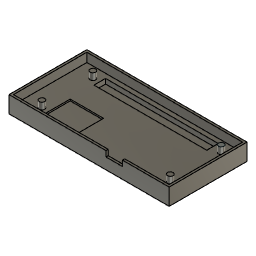
baseplate v7 (Autodesk Fusion 360 design; units mm, degrees)
Autodesk Fusion 360 part; units mm, degrees
sketch "Sketch1" plane through (0, 0, 0) normal (0, 0, 1) x (1, 0, 0)
  line L0 (0, 0) -> (70.5, 0)
  line L1 (70.5, 0) -> (70.5, 32)
  line L2 (70.5, 32) -> (0, 32)
  line L3 (0, 32) -> (0, 0)
  dimension "d1" = 70.5
  dimension "d2" = 32
  constraint horizontal L0
  constraint vertical L1
  constraint horizontal L2
  constraint vertical L3
  constraint coincident L0.start L3.end
  measures "d1" distance of L0.start L0.end
  measures "d2" distance of L0.start L2.end
extrude "Extrude1" add sketch "Sketch1" along normal blind 1.5
extrude "Extrude2" add 1 faces at (47, 32, 0.5) along direction (0, 1, 0) blind 1
extrude "Extrude3" add 1 faces at (23.5, 22, 1.5) along direction (0, 0, 1) blind 2
sketch "Sketch2" plane through (0, 0, 3.5) normal (0, 0, 1) x (-1, 0, 0)
  line L0 (0, -33) -> (0, 0)
  line L1 (0, 0) -> (-70.5, 0)
  line L2 (-70.5, 0) -> (-70.5, -33)
  line L3 (-70.5, -33) -> (0, -33)
  line L4 (-35.25, -33) -> (-35.25, -31)
  line L5 (-35.25, -31) -> (-35.25, -28.75)
  line L6 (-60.25, -26.5) -> (-10.25, -26.5)
  line L7 (-10.25, -26.5) -> (-10.25, -31)
  line L8 (-10.25, -31) -> (-60.25, -31)
  line L9 (-60.25, -31) -> (-60.25, -26.5)
  line L10 (-60.25, -26.5) -> (-10.25, -31) construction
  line L11 (-10.25, -26.5) -> (-60.25, -31) construction
  point P0 (-35.25, -28.75)
  dimension "d9" = 2
  dimension "d10" = 2.25
  dimension "d11" = 50
  dimension "d12" = 4.5
  constraint midpoint L3 L4.start
  constraint perpendicular L3 L4
  constraint perpendicular L3 L5
  constraint horizontal L6
  constraint perpendicular L6 L7
  constraint parallel L6 L8
  constraint parallel L7 L9
  constraint coincident L10 P0
  constraint coincident L11 P0
  constraint coincident P0 L5.end
  measures "d9" distance of L4.start L4.end
  measures "d10" distance of L4.end P0
  measures "d11" distance of L7.end L8.end
  measures "d12" distance of L6.end L7.end
extrude "Extrude4" cut sketch "Sketch2" against normal blind 2.2 contours L6 L7 L8 L9
extrude "Extrude5" cut 1 faces at (43.5833, 26.5, 2.7667) along direction (0, -1, 0) blind 0.7
extrude "Extrude6" cut 1 faces at (10.25, 27.5333, 2.7667) along direction (-1, 0, 0) blind 0.35
extrude "Extrude7" cut 1 faces at (60.25, 27.5333, 2.0333) along direction (1, 0, 0) blind 0.35
extrude "Extrude8" add 1 faces at (0, 22, 2.3333) along direction (-1, 0, 0) blind 1.5
extrude "Extrude9" add 1 faces at (22.5, 33, 1.1667) along direction (0, 1, 0) blind 1
extrude "Extrude10" add 1 faces at (46.5, 0, 1.1667) along direction (0, -1, 0) blind 1
sketch "Sketch3" plane through (0, 0, 3.5) normal (0, 0, 1) x (-1, 0, 0)
  line L0 (-60.6, -25.8) -> (-9.9, -25.8)
  line L1 (-9.9, -25.8) -> (-9.9, -31)
  line L2 (-9.9, -31) -> (-60.6, -31)
  line L3 (-60.6, -31) -> (-60.6, -25.8)
  line L4 (-70.5, 1) -> (-70.5, -34)
  line L5 (-70.5, -34) -> (1.5, -34)
  line L6 (1.5, -34) -> (1.5, 1)
  line L7 (1.5, 1) -> (-70.5, 1)
  line L8 (-10, -15) -> (-25, -15)
  line L9 (-25, -15) -> (-25, -3)
  line L10 (-25, -3) -> (-10, -3)
  line L11 (-10, -3) -> (-10, -15)
  constraint horizontal L8
  constraint vertical L9
  constraint horizontal L10
  constraint vertical L11
extrude "Extrude11" cut sketch "Sketch3" against normal blind 0.7 contours L8 L9 L10 L11
sketch "Sketch4" plane through (0, 0, 3.5) normal (0, 0, 1) x (-1, 0, 0)
  line L0 (-25, -15) -> (-25, -3)
  line L1 (-25, -3) -> (-10, -3)
  line L2 (-10, -3) -> (-10, -15)
  line L3 (-10, -15) -> (-25, -15)
  line L4 (-60.6, -25.8) -> (-9.9, -25.8)
  line L5 (-9.9, -25.8) -> (-9.9, -31)
  line L6 (-9.9, -31) -> (-60.6, -31)
  line L7 (-60.6, -31) -> (-60.6, -25.8)
  line L8 (-70.5, 1) -> (-70.5, -34)
  line L9 (-70.5, -34) -> (1.5, -34)
  line L10 (1.5, -34) -> (1.5, 1)
  line L11 (1.5, 1) -> (-70.5, 1)
  line L12 (1.5, -34) -> (-70.5, -34)
  line L13 (-70.5, -34) -> (-70.5, -33)
  line L14 (-70.5, -33) -> (1.5, -33)
  line L15 (1.5, -33) -> (1.5, -34)
  line L16 (1.5, 1) -> (0.5, 1)
  line L17 (0.5, 1) -> (0.5, -34)
  line L18 (0.5, -34) -> (1.5, -34)
  line L19 (1.5, -34) -> (1.5, 1)
  line L20 (1.5, 1) -> (-70.5, 1)
  line L21 (-70.5, 1) -> (-70.5, 0)
  line L22 (-70.5, 0) -> (1.5, 0)
  line L23 (1.5, 0) -> (1.5, 1)
  line L24 (-70.5, -34) -> (-69.5, -34)
  line L25 (-69.5, -34) -> (-69.5, 1)
  line L26 (-69.5, 1) -> (-70.5, 1)
  line L27 (-70.5, 1) -> (-70.5, -34)
  dimension "d29" = 1
  dimension "d30" = 1
  dimension "d31" = 1
  dimension "d32" = 1
  constraint horizontal L12
  constraint vertical L13
  constraint horizontal L14
  constraint vertical L15
  constraint coincident L9.end L10.start
  constraint horizontal L16
  constraint vertical L17
  constraint horizontal L18
  constraint vertical L19
  constraint coincident L10.end L11.start
  constraint horizontal L20
  constraint vertical L21
  constraint horizontal L22
  constraint vertical L23
  constraint horizontal L24
  constraint vertical L25
  constraint horizontal L26
  constraint vertical L27
  constraint coincident L8.end L9.start
  measures "d29" distance of L9.end L14.end
  measures "d30" distance of L10.end L16.end
  measures "d31" distance of L10.end L22.end
  measures "d32" distance of L8.end L24.end
extrude "Extrude12" add sketch "Sketch4" along normal blind 4 contours L8 L11 L20 L21 L22 L25 L26 L27 | L8 L14 L22 L25 L27 | L11 L17 L20 L22 L25 | L8 L9 L12 L13 L14 L24 L25 L27 | L10 L11 L16 L17 L19 L20 L22 L23 | L9 L12 L14 L17 L25 | L10 L14 L17 L19 L22 | L9 L10 L12 L14 L15 L17 L18 L19
sketch "Sketch5" plane through (0, 0, 3.5) normal (0, 0, 1) x (-1, 0, 0)
  line L0 (-69.5, -33) -> (0.5, -33)
  line L1 (0.5, -33) -> (0.5, 0)
  line L2 (0.5, 0) -> (-69.5, 0)
  line L3 (-69.5, 0) -> (-69.5, -33)
  line L4 (-25, -15) -> (-25, -3)
  line L5 (-25, -3) -> (-10, -3)
  line L6 (-10, -3) -> (-10, -15)
  line L7 (-10, -15) -> (-25, -15)
  line L8 (-60.6, -25.8) -> (-9.9, -25.8)
  line L9 (-9.9, -25.8) -> (-9.9, -31)
  line L10 (-9.9, -31) -> (-60.6, -31)
  line L11 (-60.6, -31) -> (-60.6, -25.8)
  line L12 (-70.5579, -29.7) -> (-66.2579, -29.7)
  circle A0 centre (-66.2579, -29.7) radius 1.375
  line L13 (-2, -34) -> (-2, -29.7)
  line L14 (1.461, -29.9433) -> (-5.539, -29.9433)
  circle A1 centre (-5.539, -29.9433) radius 1.375
  dimension "d36" = 4.3
  dimension "d37" = 2.75
  dimension "d38" = 4.3
  dimension "d39" = 7
  dimension "d40" = 2.75
  constraint perpendicular L3 L12
  constraint coincident L12.end A0.centre
  constraint perpendicular L0 L13
  constraint perpendicular L13 L14
  constraint coincident L14.end A1.centre
  measures "d36" distance of L12.start L12.end
  measures "d37" diameter of A0
  measures "d38" distance of L13.start L13.end
  measures "d39" distance of L14.start L14.end
  measures "d40" diameter of A1
extrude "Extrude13" add sketch "Sketch5" along normal blind 5 contours A0 | A1
sketch "Sketch6" plane through (0, -1, 0) normal (0, -1, 0) x (1, 0, 0)
  line L0 (-1.5, 0) -> (70.5, 0)
  line L1 (70.5, 0) -> (70.5, 7.5)
  line L2 (70.5, 7.5) -> (-1.5, 7.5)
  line L3 (-1.5, 7.5) -> (-1.5, 0)
  line L4 (70.5, 6.1254) -> (49.5, 6.1254)
  line L5 (49.5, 6.1254) -> (42.1, 6.1254)
  line L6 (42.1, 6.1254) -> (42.1, 7.5)
  line L7 (42.1, 7.5) -> (42.1, 8)
  line L8 (42.1, 8) -> (49.5, 8)
  line L9 (42.1, 8) -> (49.5, 8)
  line L10 (49.5, 8) -> (49.5, 5)
  line L11 (49.5, 5) -> (42.1, 5)
  line L12 (42.1, 5) -> (42.1, 8)
  dimension "d43" = 21
  dimension "d44" = 7.4
  dimension "d45" = 0.5
  dimension "d46" = 3
  constraint coincident L1 L4.start
  constraint perpendicular L1 L4
  constraint parallel L4 L5
  constraint coincident L2 L6.end
  constraint perpendicular L2 L6
  constraint vertical L7
  constraint perpendicular L7 L8
  constraint horizontal L9
  constraint vertical L10
  constraint horizontal L11
  constraint vertical L12
  measures "d43" distance of L4.start L4.end
  measures "d44" distance of L4.end L5.end
  measures "d45" distance of L6.end L7.end
  measures "d46" distance of L7.end L11.end
extrude "Extrude14" cut sketch "Sketch6" against normal blind 1 contours L2 L7 L8 L9 L10 L12 | L2 L5 L6 L10 L12 | L5 L10 L11 L12
sketch "Sketch7" plane through (0, 0, 3.5) normal (0, 0, 1) x (-1, 0, 0)
  circle A0 centre (-66.2579, -29.7) radius 1.375
  circle A1 centre (-5.539, -29.9433) radius 1.375
  line L0 (-69.5, -33) -> (0.5, -33)
  line L1 (0.5, -33) -> (0.5, 0)
  line L2 (0.5, 0) -> (-69.5, 0)
  line L3 (-69.5, 0) -> (-69.5, -33)
  line L4 (-25, -15) -> (-25, -3)
  line L5 (-25, -3) -> (-10, -3)
  line L6 (-10, -3) -> (-10, -15)
  line L7 (-10, -15) -> (-25, -15)
  line L8 (-60.6, -25.8) -> (-9.9, -25.8)
  line L9 (-9.9, -25.8) -> (-9.9, -31)
  line L10 (-9.9, -31) -> (-60.6, -31)
  line L11 (-60.6, -31) -> (-60.6, -25.8)
  line L12 (-66.2579, -29.7) -> (-66.2579, -6.5)
  circle A2 centre (-66.2579, -6.5) radius 1.375
  line L13 (-5.539, -29.9433) -> (-5.539, -6.7433)
  circle A3 centre (-5.539, -6.7433) radius 1.375
  dimension "d49" = 23.2
  dimension "d50" = 2.75
  dimension "d51" = 23.2
  dimension "d52" = 2.75
  constraint coincident A0.centre L12.start
  constraint parallel L3 L12
  constraint coincident L12.end A2.centre
  constraint coincident A1.centre L13.start
  constraint perpendicular L0 L13
  constraint coincident L13.end A3.centre
  measures "d49" distance of A0.centre L12.end
  measures "d50" diameter of A2
  measures "d51" distance of A1.centre L13.end
  measures "d52" diameter of A3
extrude "Extrude15" add sketch "Sketch7" along normal blind 5 contours A2 | A3
extrude "Extrude16" cut 2 faces at (66.7302, 30.022, 8.5) (66.8634, 6.1681, 8.5) along direction (0, 0, -1) blind 5
extrude "Extrude17" cut 2 faces at (5.5048, 28.9699, 8.5) (5.4119, 6.9636, 8.5) along direction (0, 0, -1) blind 5
sketch "Sketch8" plane through (0, 0, 3.5) normal (0, 0, 1) x (-1, 0, 0)
  line L0 (-69.5, -33) -> (0.5, -33)
  line L1 (0.5, -33) -> (0.5, 0)
  line L2 (0.5, 0) -> (-69.5, 0)
  line L3 (-69.5, 0) -> (-69.5, -33)
  line L4 (-25, -15) -> (-25, -3)
  line L5 (-25, -3) -> (-10, -3)
  line L6 (-10, -3) -> (-10, -15)
  line L7 (-10, -15) -> (-25, -15)
  line L8 (-60.6, -25.8) -> (-9.9, -25.8)
  line L9 (-9.9, -25.8) -> (-9.9, -31)
  line L10 (-9.9, -31) -> (-60.6, -31)
  line L11 (-60.6, -31) -> (-60.6, -25.8)
  line L12 (-70.5, -34) -> (-70.5, -28.2)
  line L13 (-70.5, -28.2) -> (-66.5, -28.2)
  line L14 (-70.5, -34) -> (-64.7, -34)
  line L15 (-64.7, -34) -> (-64.7, -30)
  line L16 (-64.7, -30) -> (-64.7, -27.5)
  line L17 (-66.5, -28.2) -> (-64.7, -28.2)
  circle A0 centre (-64.7, -28.2) radius 1.25
  line L18 (-64.7, -28.2) -> (-64.7, -26.95)
  line L19 (-64.7, -26.95) -> (-64.7, -6.95)
  circle A1 centre (-64.7, -5.7) radius 1.25
  line L20 (-64.7, -5.7) -> (-8.25, -5.7)
  circle A2 centre (-7, -5.7) radius 1.25
  line L21 (-7, -5.7) -> (-7, -26.95)
  circle A3 centre (-7, -28.2) radius 1.25
  dimension "d72" = 5.8
  dimension "d74" = 4
  dimension "d75" = 5.8
  dimension "d76" = 4
  dimension "d77" = 2.5
  dimension "d78" = 1.25
  dimension "d79" = 20
  dimension "d80" = 2.5
  dimension "d81" = 56.45
  dimension "d82" = 2.5
  dimension "d83" = 21.25
  dimension "d84" = 2.5
  constraint perpendicular L0 L12
  constraint perpendicular L12 L13
  constraint perpendicular L12 L14
  constraint perpendicular L0 L15
  constraint parallel L15 L16
  constraint coincident L16 L17.end
  constraint perpendicular L16 L17
  constraint coincident L17.end A0.centre
  constraint perpendicular L17 L18
  constraint parallel L18 L19
  constraint coincident L19.end A1
  constraint coincident A1.centre L20.start
  constraint perpendicular L3 L20
  constraint coincident L20.end A2
  constraint coincident A2.centre L21.start
  constraint parallel L1 L21
  constraint coincident L21.end A3
  measures "d72" distance of L12.start L12.end
  measures "d74" distance of L12.end L13.end
  measures "d75" distance of L12.start L14.end
  measures "d76" distance of L14.end L15.end
  measures "d77" diameter of A0
  measures "d78" distance of L17.end L18.end
  measures "d79" distance of L18.end L19.end
  measures "d80" diameter of A1
  measures "d81" distance of A1.centre L20.end
  measures "d82" diameter of A2
  measures "d83" distance of A2.centre L21.end
  measures "d84" diameter of A3
extrude "Extrude18" add sketch "Sketch8" along normal blind 3 contours L16 L17 A0 | L16 A0 L18 | L16 L17 A0 L18 | A1 | A2 | A3
sketch "Sketch9" plane through (0, 0, 6.5) normal (0, 0, 1) x (-1, 0, 0)
  circle A0 centre (-64.7, -28.2) radius 1.25
extrude "Extrude19" cut 2 faces at (6.88, 5.4166, 6.5) (64.5007, 5.6393, 6.5) along direction (0, 0, -1) blind 3
sketch "Sketch10" plane through (0, 0, 3.5) normal (0, 0, 1) x (-1, 0, 0)
  circle A0 centre (-64.7, -28.2) radius 1.25
  circle A1 centre (-7, -28.2) radius 1.25
  line L0 (-69.5, -33) -> (0.5, -33)
  line L1 (0.5, -33) -> (0.5, 0)
  line L2 (0.5, 0) -> (-69.5, 0)
  line L3 (-69.5, 0) -> (-69.5, -33)
  line L4 (-25, -15) -> (-25, -3)
  line L5 (-25, -3) -> (-10, -3)
  line L6 (-10, -3) -> (-10, -15)
  line L7 (-10, -15) -> (-25, -15)
  line L8 (-60.6, -25.8) -> (-9.9, -25.8)
  line L9 (-9.9, -25.8) -> (-9.9, -31)
  line L10 (-9.9, -31) -> (-60.6, -31)
  line L11 (-60.6, -31) -> (-60.6, -25.8)
  line L12 (-64.7, -28.2) -> (-64.7, -26.95)
  line L13 (-64.7, -26.95) -> (-64.7, -6.55)
  circle A2 centre (-64.7, -5.3) radius 1.25
  line L14 (-64.7, -5.3) -> (-63.45, -5.3)
  line L15 (-63.45, -5.3) -> (-8.25, -5.3)
  circle A3 centre (-7, -5.3) radius 1.25
  dimension "d89" = 20.4
  dimension "d90" = 2.5
  dimension "d91" = 55.2
  dimension "d92" = 2.5
  constraint coincident A0.centre L12.start
  constraint coincident A0 L12.end
  constraint parallel L11 L12
  constraint parallel L12 L13
  constraint coincident L13.end A2
  constraint coincident A2.centre L14.start
  constraint coincident A2 L14.end
  constraint parallel L2 L14
  constraint parallel L14 L15
  constraint coincident L15.end A3
  measures "d89" distance of L12.end L13.end
  measures "d90" diameter of A2
  measures "d91" distance of L14.end L15.end
  measures "d92" diameter of A3
extrude "Extrude20" add sketch "Sketch10" along normal blind 3 contours A2 | A3
